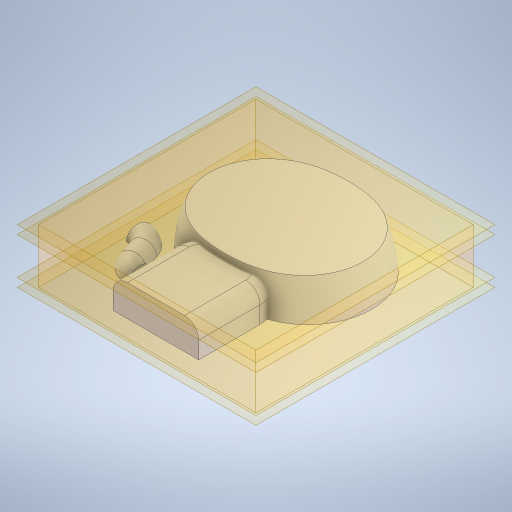
# Autodesk Inventor part: MOLDE
Saved by Autodesk Inventor 2023.2 (Build 272271030, 271C)
## iProperties
Created: 2023-08-26
Part Number: MOLDE
Material: Generic
Document SubType Name: Modeling
Designer: Cris Pat
Density: 1 g/cm^3
Appearance: Default
Author: Cris Pat
Autodesk Inventor part; units mm, degrees
ref_plane "YZ Plane" through (0, 0, 0) normal (1, 0, 0) x (0, 1, 0)
ref_plane "XZ Plane" through (0, 0, 0) normal (0, 1, 0) x (-1, 0, 0)
sketch "Sketch1" plane through (0, 0, 0) normal (0, 0, 1) x (1, 0, 0)
  line L0 (0, 76.2) -> (76.2, 76.2)
  line L1 (76.2, 76.2) -> (76.2, 0)
  line L2 (76.2, 0) -> (0, 0)
  line L3 (0, 0) -> (0, 76.2)
  dimension "d0" = 76.2
  dimension "d1" = 76.2
  constraints: 8 end point, 2 parallel, 1 coincident, 1 horizontal, 1 perpendicular
  measures "d0" distance between parallel lines of L1 L3
  measures "d1" distance between parallel lines of L2 L0
surface extrude "STOCK_LIMITE_PERIMETRAL" sketch "Sketch1" against normal blind 19.05 shown yes curves L3 L0 L1 L2
ref_plane "STOCK_LIMITE_INFERIOR" through (0, 0, -19.05) normal (0, 0, 1) x (1, 0, 0)
ref_plane "PIEZA_LIMITE_SUPERIOR" through (0, 0, -3) normal (0, 0, 1) x (1, 0, 0)
ref_plane "PIEZA_LIMITE_INFERIOR" through (0, 0, -16.05) normal (0, 0, 1) x (1, 0, 0)
sketch "Sketch2" plane through (0, 0, -16.05) normal (0, 0, 1) x (1, 0, 0)
  line L0 (0, 76.2) -> (76.2, 76.2) construction
  line L1 (76.2, 0) -> (0, 0) construction
  line L2 (0, 0) -> (0, 76.2) construction
  line L3 (76.2, 76.2) -> (76.2, 0) construction
  line L4 (6.6, 71.2) -> (69.6, 71.2)
  line L5 (69.6, 71.2) -> (69.6, 26.2)
  line L6 (69.6, 26.2) -> (6.6, 26.2)
  line L7 (6.6, 26.2) -> (6.6, 71.2)
  line L8 (0, 76.2) -> (76.2, 76.2) construction
  point P0 (38.1, 71.2)
  point P1 (38.1, 76.2)
  point P2 (38.1, 76.2)
  dimension "d7" = 45
  dimension "d8" = 63
  dimension "d9" = 5
  constraints: 8 end point, 3 midpoint, 2 parallel, 1 horizontal, 1 perpendicular, 1 vertical alignment
  measures "d7" distance between parallel lines of L6 L4
  measures "d8" distance between parallel lines of L5 L7
  measures "d9" distance of point (38.1, 71.2) point (38.1, 76.2)
extrude "Extrusion1" add sketch "Sketch2" along normal up to surface (13.05 mm away)
fillet "Fillet1" [suppressed]
sketch "Sketch5" plane through (0, 0, -16.05) normal (0, 0, 1) x (1, 0, 0)
  line L0 (6.6, 26.2) -> (6.6, 71.2) construction
  line L1 (69.6, 26.2) -> (6.6, 26.2) construction
  line L2 (69.6, 71.2) -> (69.6, 26.2) construction
  line L3 (6.6, 71.2) -> (69.6, 71.2) construction
  line L4 (38.1, 71.2) -> (38.1, 26.2)
  arc A0 (45.6, 26.2) -> (45.6, 71.2) centre (45.6, 48.7) ccw
  line L5 (45.6, 71.2) -> (38.1, 71.2)
  line L6 (45.6, 26.2) -> (38.1, 26.2)
  point P0 (0, 0)
  point P1 (38.1, 48.7)
  point P2 (68.1, 48.7)
  dimension "d21" = 30
  constraints: 6 end point, 3 midpoint, 3 point on circle, 2 collinear, 2 point on line, 2 tangent, 1 centre point, 1 coincident
  measures "d21" distance of point (38.1, 48.7) point (68.1, 48.7)
revolve "Revolution3" cut sketch "Sketch5" angle 180 about axis through (38.1, 71.2, -16.05) along (0, -1, 0) keep common part
sketch "Sketch6" plane through (0, 0, -16.05) normal (0, 0, 1) x (1, 0, 0)
  arc A0 (30.6, 71.2) -> (30.6, 26.2) centre (30.6, 48.7) ccw construction
  line L0 (45.6, 71.2) -> (30.6, 71.2) construction
  arc A1 (45.6, 26.2) -> (45.6, 71.2) centre (45.6, 48.7) ccw construction
  line L1 (0, 76.2) -> (76.2, 76.2) construction
  line L2 (76.2, 0) -> (0, 0) construction
  line L3 (23.1, 34.5) -> (53.1, 34.5)
  line L4 (53.1, 34.5) -> (53.1, 3)
  line L5 (53.1, 3) -> (23.1, 3)
  line L6 (23.1, 3) -> (23.1, 34.5)
  point P0 (38.1, 34.5)
  point P1 (38.1, 0)
  dimension "d23" = 30
  dimension "d24" = 31.5
  dimension "d25" = 3
  constraints: 8 end point, 2 midpoint, 2 parallel, 1 horizontal, 1 perpendicular, 1 vertical alignment, 1 other
  measures "d23" distance between parallel lines of L4 L6
  measures "d24" distance between parallel lines of L5 L3
  measures "d25" distance between parallel lines of L2 L5
extrude "Extrusion2" add sketch "Sketch6" along normal blind 11 separate body
fillet "Fillet2" radius 10 2 edges at (23.1, 34.5, -10.55) (53.1, 34.5, -10.55)
fillet "Fillet3" radius 5 5 edges at (26.0289, 31.5711, -5.05) (38.1, 34.5, -5.05) (50.1711, 31.5711, -5.05) (53.1, 13.75, -5.05) (23.1, 13.75, -5.05)
sketch "Sketch9" plane through (23.1, 3, -16.05) normal (-1, 0, 0) x (0, 0, 1)
  line L0 (6, 21.5) -> (6, 0) construction
  line L1 (0, 21.5) -> (6, 21.5) construction
  line L2 (0, 21.5) -> (0, 0) construction
  line L3 (0, 0) -> (6, 0) construction
  arc A0 (0, 11.5) -> (0, 19.5) centre (0, 15.5) ccw
  line L4 (0, 19.5) -> (0, 11.5)
  point P0 (16.05, -3)
  dimension "d37" = 2
  dimension "d45" = 4
  constraints: 2 end point, 2 point on circle, 2 vertical alignment, 1 centre point, 1 collinear, 1 point on line
  measures "d37" distance of L4.start L1.start
  measures "d45" radius of A0
sketch "Sketch10" plane through (0, 0, -16.05) normal (0, 0, 1) x (1, 0, 0)
  line L0 (23.1, 18.5) -> (18.1, 17.5)
  arc A0 (12.4096, 20.5) -> (18.1, 17.5) centre (17.1, 22.5) ccw
  point P0 (0, 0)
  dimension "d47" = 1
  dimension "d48" = 6
  dimension "d50" = 2
  dimension "d51" = 4
  constraints: 2 end point, 2 point on circle, 1 centre point, 1 tangent
  measures "d47" vertical distance of L0.start L0.end
  measures "d48" horizontal distance of L0.start A0.centre
  measures "d50" vertical distance of A0.start A0.centre
  measures "d51" vertical distance of L0.start A0.centre
sweep "Sweep1" add profiles "Sketch9" path "Sketch10" separate body
sketch "Sketch11" plane through (12.4096, 20.5, -16.05) normal (-0.2042148, 0.9789261, 0) x (0.9789261, 0.2042148, 0)
  line L0 (4.141, 0) -> (-4, 0) construction
  arc A0 (-4, 0) -> (4, 0) centre (0, 0) ccw
  line L1 (4, 0) -> (-4, 0)
  line L2 (9.2398, 0) -> (4.141, 0) construction
  point P0 (-16.3345, -16.05)
  dimension "d54" = 4
  constraints: 2 end point, 2 point on circle, 1 centre point, 1 collinear, 1 horizontal alignment
  measures "d54" radius of A0
sketch "Sketch12" plane through (0, 0, -16.05) normal (0, 0, 1) x (1, 0, 0)
  line L0 (12.4096, 20.5) -> (10.4742, 26.1793)
  arc A0 (10.4742, 26.1793) -> (5.1048, 30.1586) centre (4.9096, 24.283) ccw
  line L1 (16.3253, 21.3169) -> (8.4939, 19.6831) projected
  point P0 (0, 0)
  point P1 (12.4096, 20.5)
  dimension "d55" = 6
  dimension "d56" = 7.5
  dimension "d57" = 3.783
  dimension "d58" = 5.8756
  constraints: 2 end point, 2 point on circle, 1 centre point, 1 midpoint, 1 tangent
  measures "d55" distance of L0.start L0.end
  measures "d56" horizontal distance of A0.centre L0.start
  measures "d57" vertical distance of point (12.41, 20.5) A0.centre
  measures "d58" vertical distance of A0.centre A0.end
sweep "Sweep2" add profiles "Sketch11" path "Sketch12" separate body path curves L0 A0
equation "\"d8\" = 1.4 * d7"
equation "\"d24\" = 1.05 * d23"
body "Solid1"
body "Srf1"
body "Solid2"
body "Solid4"
body "Solid5"
